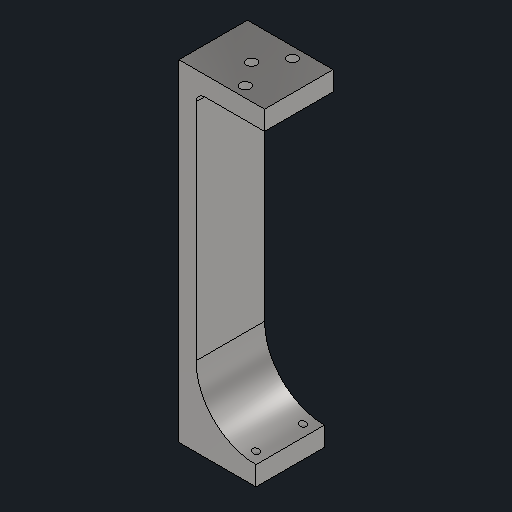
# Autodesk Inventor part: KN-00-02-09
Saved by Autodesk Inventor 2025.2 (Build 292293000, 293)
## iProperties
Created: 2025-04-22
Part Number: KN-00-02-09
Material: X5CrNi18-10
Document SubType Name: Modeling
Designer: Kacper Mik
Density: 8 g/cm^3
Appearance: Semi-Polished
Mass: 61.6621 g
Surface Area: 45.7372 cm^2
Volume: 7.70777 cm^3
Author: Kacper Mik
Autodesk Inventor part; units mm, degrees
ref_plane "YZ Plane" through (0, 0, 0) normal (1, 0, 0) x (0, 1, 0)
ref_plane "XZ Plane" through (0, 0, 0) normal (0, 1, 0) x (-1, 0, 0)
sketch "Sketch1" plane through (0, 0, 0) normal (0, 1, 0) x (-1, 0, 0)
  line L0 (9, 8) -> (-9, 8)
  line L1 (-9, 8) -> (-9, -8)
  line L2 (-9, -8) -> (9, -8)
  line L3 (9, -8) -> (9, 8)
  line L4 (9, 8) -> (-9, -8) construction
  line L5 (-9, 8) -> (9, -8) construction
  point P0 (0, 0)
  dimension "d0" = 18
  dimension "d1" = 16
  constraints: 12 end point, 2 midpoint, 2 parallel, 1 horizontal, 1 perpendicular
  measures "d0" distance of L2.end L1.end
  measures "d1" distance of L1.end L0.end
extrude "Extrusion1" add sketch "Sketch1" along normal blind 4.5
ref_plane "Work Plane1" through (-12, 77.38, -8) normal (0, -1, 0) x (1, 0, 0)
sketch "Sketch6" plane through (0, 4.5, 0) normal (0, 1, 0) x (1, 0, 0)
  line L0 (9, 8) -> (-9, 8) projected
  line L1 (-9, -8) -> (9, -8) projected
  line L2 (-9, 8) -> (-5, 8)
  line L3 (-5, 8) -> (-5, -8)
  line L4 (-5, -8) -> (-9, -8)
  line L5 (-9, -8) -> (-9, 8)
  line L6 (9, -8) -> (9, 8) projected
  point P0 (0, 0)
  dimension "d27" = 14
  constraints: 8 end point, 2 parallel, 1 horizontal, 1 perpendicular, 1 point on line
  measures "d27" distance between parallel lines of L3 L6
extrude "WAZNE" add sketch "Sketch6" along normal up to surface (72.88 mm away) contours L3 L1 L5 L0
fillet "Fillet2" radius 14 1 edges at (-5, 4.5, 0)
sketch "Sketch7" plane through (0, 0, 0) normal (0, -1, 0) x (1, 0, 0)
  line L0 (-4.5, 5.5) -> (6.5, 5.5) construction
  line L1 (6.5, 5.5) -> (6.5, -5.5) construction
  line L2 (6.5, -5.5) -> (-4.5, -5.5) construction
  line L3 (-4.5, -5.5) -> (-4.5, 5.5) construction
  line L4 (9, 8) -> (9, -8) projected
  line L5 (-9, 8) -> (9, 8) projected
  point P0 (0, 0)
  dimension "d31" = 11
  dimension "d32" = 11
  dimension "d33" = 2.5
  dimension "d34" = 2.5
  constraints: 8 end point, 4 coincident, 2 parallel, 1 horizontal, 1 perpendicular
  measures "d31" distance of L0.start L0.end
  measures "d32" distance of L0.end L1.end
  measures "d33" distance from line of L4 point (6.5, 5.5)
  measures "d34" distance from line of L5 point (6.5, 5.5)
hole "Hole2" at (6.5, 0, 5.5) at (-4.5, 0, 5.5) at (-4.5, 0, -5.5) at (6.5, 0, -5.5) direction (0, 1, 0) diameter 1.567 depth 5.5 thread size "M2x0.4" class "6H" standard "ISO Metric profile"
chamfer "Chamfer2" distance 0.2 angle 45 4 edges at (-4.5, 0, 6.2835) (6.5, 0, 6.2835) (6.5, 0, -4.7165) (-4.5, 0, -4.7165)
sketch "Sketch8" plane through (0, 77.38, 0) normal (0, 1, 0) x (1, 0, 0)
  line L0 (-9, 8) -> (-9, -8) projected
  line L1 (11, -8) -> (11, 8)
  line L2 (-9, 8) -> (11, 8)
  line L3 (11, 8) -> (11, -8)
  line L4 (11, -8) -> (-9, -8)
  line L5 (-9, -8) -> (-9, 8)
  point P0 (0, 0)
  point P1 (11, 8)
  dimension "d63" = 20
  constraints: 10 end point, 2 parallel, 1 horizontal, 1 perpendicular
  measures "d63" distance of L1.start L4.end
extrude "Extrusion6" add sketch "Sketch8" against normal blind 4.5
sketch "Sketch9" plane through (0, 72.88, 0) normal (0, -1, 0) x (1, 0, 0)
  line L0 (11, 8) -> (11, -8) projected
  line L1 (-5, -8) -> (-5, 8) projected
  line L2 (4, 7.0265) -> (4, -6.0756) construction
  point P0 (0, 0)
  point P1 (0, 0)
  point P2 (4, 5.5)
  point P3 (4, -5.5)
  dimension "d52" = 5
  dimension "d67" = 7
  dimension "d68" = 4
  dimension "d69" = 11
  dimension "d70" = 5.5
  constraints: 2 end point, 2 point on line, 1 coincident, 1 vertical
  measures "d52" distance from line of L1 point (0, 0)
  measures "d67" distance between parallel lines of L0 L2
  measures "d68" distance from line of L2 point (0, 0)
  measures "d69" distance of point (4, -5.5) point (4, 5.5)
  measures "d70" vertical distance of point (4, 5.5) point (0, 0)
hole "Hole3" at (0, 72.88, 0) at (4, 72.88, 5.5) at (4, 72.88, -5.5) direction (0, 1, 0) diameter 2.4 end through all clearance for "Countersunk Flat Head Screw ISO 2009/7046" size "M2" standard "ISO"
chamfer "Chamfer3" distance 0.2 angle 45 3 edges at (0, 72.88, 1.2) (4, 72.88, 6.7) (4, 72.88, -4.3)
fillet "Fillet4" radius 2 1 edges at (-5, 72.88, 0)
equation "\"d70\" = 0.5 * d69"
body "Solid1"
